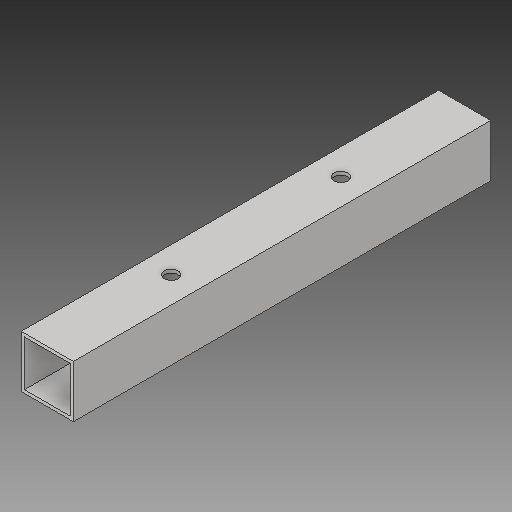
# Autodesk Inventor part: AlumBracket1x1
Saved by Autodesk Inventor 2019.3 (Build 233278000, 278)
## iProperties
Created: 2018-12-25
Part Number: AlumBracket1x1
Material: Generic
Document SubType Name: Modeling
Designer: steele
Density: 1 g/cm^3
Appearance: Default
Author: steele
Autodesk Inventor part; units mm, degrees
ref_plane "YZ Plane" through (0, 0, 0) normal (1, 0, 0) x (0, 1, 0)
ref_plane "XZ Plane" through (0, 0, 0) normal (0, 1, 0) x (-1, 0, 0)
ref_plane "XY Plane" through (0, 0, 0) normal (0, 0, 1) x (1, 0, 0)
sketch "Sketch1" plane through (0, 0, 0) normal (0, 0, 1) x (1, 0, 0)
  line L0 (-12.7, -12.7) -> (12.7, -12.7)
  line L1 (12.7, -12.7) -> (12.7, 12.7)
  line L2 (12.7, 12.7) -> (-12.7, 12.7)
  line L3 (-12.7, 12.7) -> (-12.7, -12.7)
  line L4 (-12.7, -12.7) -> (12.7, 12.7) construction
  line L5 (12.7, -12.7) -> (-12.7, 12.7) construction
  line L6 (-11.1125, -11.1125) -> (11.1125, -11.1125)
  line L7 (11.1125, -11.1125) -> (11.1125, 11.1125)
  line L8 (11.1125, 11.1125) -> (-11.1125, 11.1125)
  line L9 (-11.1125, 11.1125) -> (-11.1125, -11.1125)
  line L10 (-11.1125, -11.1125) -> (11.1125, 11.1125) construction
  line L11 (11.1125, -11.1125) -> (-11.1125, 11.1125) construction
  point P0 (0, 0)
  dimension "d0" = 25.4
  dimension "d1" = 25.4
  dimension "d2" = 22.225
  constraints: 24 end point, 4 midpoint, 4 parallel, 3 perpendicular, 2 horizontal
  measures "d0" distance of L0.start L0.end
  measures "d1" distance of L1.end L0.end
  measures "d2" distance of L6.start L6.end
extrude "Extrusion1" add sketch "Sketch1" along normal mid plane 203.2
sketch "Sketch4" plane through (-12.7, 12.7, 101.6) normal (0, 1, 0) x (1, 0, 0)
  point P0 (12.7, 60.325)
  point P1 (12.7, 142.875)
hole "Hole4" at (0, 12.7, 41.275) at (0, 12.7, -41.275) direction (0, -1, 0) diameter 6.7564 depth 1.5875
sketch "Sketch5" plane through (-11.1125, -11.1125, -101.6) normal (0, 1, 0) x (1, 0, 0)
  point P0 (11.1125, -142.875)
  point P1 (11.1125, -60.325)
hole "Hole6" at (0, -11.1125, 41.275) at (0, -11.1125, -41.275) direction (0, -1, 0) diameter 6.7564 depth 1.5875
body "Solid1"
